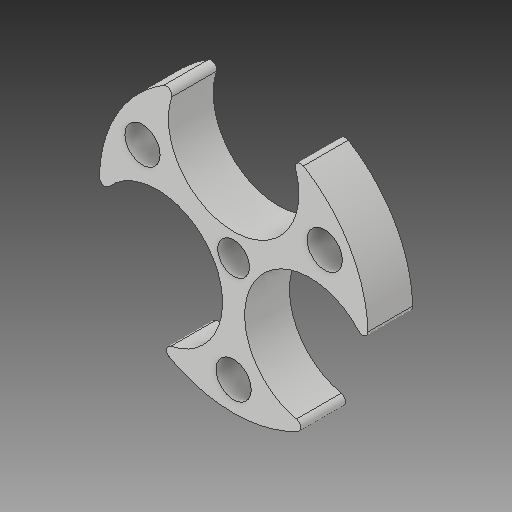
# Autodesk Inventor part: battery_holder
Saved by Autodesk Inventor 2018.1 (Build 221171000, 171)
## iProperties
Created: 2017-08-10
Part Number: battery_holder
Material: Generic
Document SubType Name: Modeling
Designer: Kai
Density: 1 g/cm^3
Appearance: Default
Author: Kai
Autodesk Inventor part; units mm, degrees
ref_plane "YZ Plane" through (0, 0, 0) normal (1, 0, 0) x (0, 1, 0)
ref_plane "XZ Plane" through (0, 0, 0) normal (0, 1, 0) x (-1, 0, 0)
ref_plane "XY Plane" through (0, 0, 0) normal (0, 0, 1) x (1, 0, 0)
sketch "Sketch1" plane through (0, 0, 0) normal (0, 0, 1) x (1, 0, 0)
  circle A0 centre (0, 0) radius 12.5 construction
  arc A1 (-7.8805, 17.3436) -> (7.8805, 17.3436) centre (0, 12.5) ccw
  arc A2 (-11.0798, -15.4965) -> (-18.9602, -1.8471) centre (-10.8253, -6.25) ccw
  arc A3 (18.9602, -1.8471) -> (11.0798, -15.4965) centre (10.8253, -6.25) ccw
  arc A4 (-7.8805, 17.3436) -> (-18.9602, -1.8471) centre (0, 0) ccw
  arc A5 (-11.0798, -15.4965) -> (11.0798, -15.4965) centre (0, 0) ccw
  arc A6 (18.9602, -1.8471) -> (7.8805, 17.3436) centre (0, 0) ccw
  dimension "d0" = 25
  dimension "d1" = 18.5
  dimension "d5" = 360
  constraints: 12 point on circle, 6 centre point, 2 coincident, 1 vertical alignment, 15 other
  measures "d1" diameter of A1
extrude "Extrusion1" add sketch "Sketch1" along normal blind 6.35
fillet "Fillet1" radius 0.762 6 edges at (-7.8805, 17.3436, 3.175) (7.8805, 17.3436, 3.175) (18.9602, -1.8471, 3.175) (11.0798, -15.4965, 3.175) (-11.0798, -15.4965, 3.175) (-18.9602, -1.8471, 3.175)
sketch "Sketch2" plane through (0, 0, 6.35) normal (0, 0, 1) x (1, 0, 0)
  circle A0 centre (0, 0) radius 14.9225 construction
  circle A1 centre (0, -14.9225) radius 2.5
  circle A2 centre (12.9233, 7.4612) radius 2.5
  circle A3 centre (-12.9233, 7.4613) radius 2.5
  dimension "d10" = 29.845
  dimension "d11" = 5
  dimension "d14" = 360
  constraints: 3 centre point, 1 coincident, 1 vertical alignment, 9 other
  measures "d11" diameter of A1
extrude "Extrusion2" cut sketch "Sketch2" against normal blind 6.35
sketch "Sketch3" plane through (0, 0, 6.35) normal (0, 0, 1) x (1, 0, 0)
  circle A0 centre (0, 0) radius 2.25
  dimension "d18" = 4.5
  constraints: 1 centre point, 1 coincident
  measures "d18" diameter of A0
extrude "Extrusion3" cut sketch "Sketch3" against normal blind 6.35
body "Solid1"
